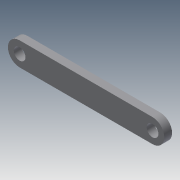
# Autodesk Inventor part: neco3
Saved by Autodesk Inventor 2013 (Build 170138000, 138)
## iProperties
Created: 2013-03-09
Part Number: neco3
Material: Generic
Document SubType Name: Modeling
Designer: idle-rug
Density: 1 g/cm^3
Author: idle-rug
Autodesk Inventor part; units mm, degrees
ref_plane "YZ Plane" through (0, 0, 0) normal (1, 0, 0) x (0, 1, 0)
ref_plane "XZ Plane" through (0, 0, 0) normal (0, 1, 0) x (-1, 0, 0)
ref_plane "XY Plane" through (0, 0, 0) normal (0, 0, 1) x (1, 0, 0)
sketch "Sketch1" plane through (0, 0, 0) normal (0, 1, 0) x (-1, 0, 0)
  line L0 (-17, -3) -> (17, -3)
  line L1 (17, -3) -> (17, 3)
  line L2 (17, 3) -> (-17, 3)
  line L3 (-17, 3) -> (-17, -3)
  line L4 (-17, -3) -> (17, 3) construction
  line L5 (17, -3) -> (-17, 3) construction
  circle A0 centre (17, 0) radius 3
  circle A1 centre (-17, 0) radius 3
  point P0 (0, 0)
  dimension "d0" = 34
  dimension "d1" = 6
  constraints: 12 end point, 4 midpoint, 2 parallel, 2 vertical alignment, 1 horizontal, 1 perpendicular, 4 other
  measures "d0" distance of L2.end L1.end
  measures "d1" distance of L1.end L0.end
extrude "Extrusion1" add sketch "Sketch1" along normal blind 2
sketch "Sketch2" plane through (0, 2, 0) normal (0, 1, 0) x (1, 0, 0)
  arc A0 (17, -3) -> (17, 3) centre (17, 0) ccw projected
  arc A1 (-17, 3) -> (-17, -3) centre (-17, 0) ccw projected
  circle A2 centre (-17, 0) radius 1.5
  circle A3 centre (17, 0) radius 1.5
  point P0 (0, 0)
  dimension "d4" = 3
  dimension "d5" = 3
  constraints: 2 centre point, 2 coincident
  measures "d4" diameter of A2
  measures "d5" diameter of A3
extrude "Extrusion2" cut sketch "Sketch2" against normal blind 2
body "Solid1"
